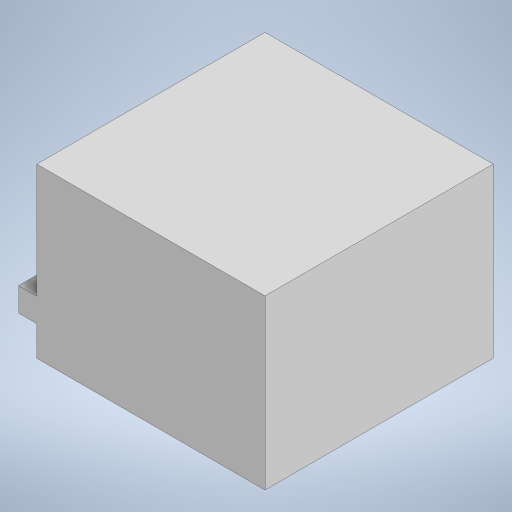
# Autodesk Inventor part: ReadArduinoHolder
Saved by Autodesk Inventor 2024 (Build 280153000, 153)
## iProperties
Created: 2023-07-12
Part Number: ReadArduinoHolder
Material: Generic
Document SubType Name: Modeling
Designer: thoma
Density: 1 g/cm^3
Appearance: Default
Author: thoma
Autodesk Inventor part; units mm, degrees
ref_plane "YZ Plane" through (0, 0, 0) normal (1, 0, 0) x (0, 1, 0)
ref_plane "XZ Plane" through (0, 0, 0) normal (0, 1, 0) x (-1, 0, 0)
ref_plane "XY Plane" through (0, 0, 0) normal (0, 0, 1) x (1, 0, 0)
sketch "Sketch1" plane through (0, 0, 0) normal (0, 1, 0) x (-1, 0, 0)
  line L0 (4.2133, 10.4249) -> (-14.7867, 10.4249)
  line L1 (-14.7867, 10.4249) -> (-14.7867, -8.5751)
  line L2 (-14.7867, -8.5751) -> (4.2133, -8.5751)
  line L3 (4.2133, -8.5751) -> (4.2133, 10.4249)
  point P0 (0, 0)
  dimension "d0" = 19
  dimension "d1" = 19
  constraints: 8 end point, 2 parallel, 1 horizontal, 1 perpendicular
  measures "d0" distance of L2.end L0.start
  measures "d1" distance of L0.start L0.end
extrude "Extrusion1" add sketch "Sketch1" along normal blind 14
sketch "Sketch2" plane through (-4.2133, 0, -8.5751) normal (-1, 0, 0) x (0, 0, 1)
  line L0 (0, 0) -> (0, 14) projected
  line L1 (19, 0) -> (19, 14) projected
  line L2 (0, 4.5) -> (19, 4.5)
  line L3 (19, 4.5) -> (19, 2.5)
  line L4 (19, 2.5) -> (0, 2.5)
  line L5 (0, 2.5) -> (0, 4.5)
  line L6 (0, 0) -> (19, 0) projected
  point P0 (8.5751, 0)
  point P1 (0, 2.5)
  dimension "d4" = 2
  dimension "d5" = 2.5
  constraints: 8 end point, 2 parallel, 2 point on line, 1 horizontal, 1 perpendicular
  measures "d4" distance between parallel lines of L4 L2
  measures "d5" distance between parallel lines of L6 L4
extrude "Extrusion2" add sketch "Sketch2" along normal blind 1.5 contours L0 L2 L1 L4
body "Solid1"
